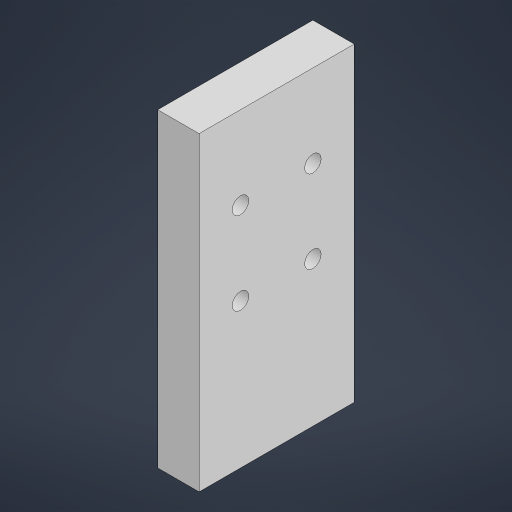
# Autodesk Inventor part: BallSensor_Mount
Saved by Autodesk Inventor 2024.2 (Build 282272000, 272)
## iProperties
Created: 2023-12-21
Part Number: BallSensor_Mount
Material: 一般
Document SubType Name: Modeling
Designer: Hanaoka
Density: 1 g/cm^3
Appearance: 既定
Author: Hanaoka
Autodesk Inventor part; units mm, degrees
ref_plane "YZ Plane" through (0, 0, 0) normal (1, 0, 0) x (0, 1, 0)
ref_plane "XZ Plane" through (0, 0, 0) normal (0, 1, 0) x (-1, 0, 0)
ref_plane "XY Plane" through (0, 0, 0) normal (0, 0, 1) x (1, 0, 0)
sketch "スケッチ1" plane through (0, 0, 0) normal (0, 1, 0) x (-1, 0, 0)
  line L0 (-2, 7.5) -> (2, 7.5)
  line L1 (2, 7.5) -> (2, -7.5)
  line L2 (2, -7.5) -> (-2, -7.5)
  line L3 (-2, -7.5) -> (-2, 7.5)
  line L4 (-2, 7.5) -> (2, -7.5) construction
  line L5 (2, 7.5) -> (-2, -7.5) construction
  circle A0 centre (0, 5.5) radius 1
  circle A1 centre (0, -5.5) radius 1
  line L6 (0, 5.5) -> (0, 7.5) construction
  line L7 (0, -5.5) -> (0, -7.5) construction
  point P0 (0, 0)
  dimension "d0" = 4
  dimension "d1" = 15
  dimension "d2" = 2
  dimension "d3" = 2
  constraints: 16 end point, 4 midpoint, 2 centre point, 2 parallel, 2 vertical, 1 collinear, 1 equal radius, 1 horizontal, 1 perpendicular
  measures "d0" distance of L1.end L2.end
  measures "d1" distance of L0.end L1.end
  measures "d2" diameter of A0
  measures "d3" distance of L6.start L6.end
extrude "押し出し1" add sketch "スケッチ1" along normal blind 30 contours L0 L1 L2 L3 | A0 | A1
extrude "押し出し2" cut sketch "スケッチ1" along normal blind 6 contours A0 | A1
sketch "スケッチ2" plane through (-2, 0, -7.5) normal (-1, 0, 0) x (0, 0, 1)
  line L0 (4, 12) -> (11, 12)
  line L1 (13, 14) -> (13, 22)
  line L2 (11, 24) -> (4, 24)
  line L3 (2, 22) -> (2, 14)
  arc A0 (2, 14) -> (4, 12) centre (4, 14) ccw
  arc A1 (4, 24) -> (2, 22) centre (4, 22) ccw
  arc A2 (13, 22) -> (11, 24) centre (11, 22) ccw
  arc A3 (11, 12) -> (13, 14) centre (11, 14) ccw
  line L4 (7.5, 0) -> (7.5, 30) construction
  line L5 (0, 30) -> (15, 30) projected
  circle A4 centre (4, 14) radius 0.8
  circle A5 centre (4, 22) radius 0.8
  circle A6 centre (11, 22) radius 0.8
  circle A7 centre (11, 14) radius 0.8
  point P0 (2, 12)
  point P1 (13, 24)
  point P2 (2, 24)
  dimension "d8" = 12
  dimension "d9" = 11
  dimension "d10" = 2
  dimension "d11" = 6
  dimension "d12" = 1.6
  constraints: 10 end point, 8 centre point, 8 point on circle, 8 tangent, 6 equal radius, 6 point on line, 4 coincident, 2 parallel, 1 horizontal, 1 midpoint, 1 perpendicular, 1 vertical, 1 other
  measures "d8" distance of point (2, 24) point (2, 12)
  measures "d9" distance of point (13, 24) point (2, 24)
  measures "d10" radius of A0
  measures "d11" distance between parallel lines of L5 L2
  measures "d12" diameter of A4
extrude "押し出し3" cut sketch "スケッチ2" against normal blind 1
extrude "押し出し4" cut sketch "スケッチ2" against normal up to surface (4 mm away) contours A4 | A5 | A6 | A7
